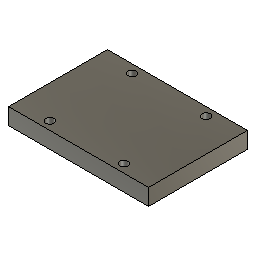
Top (Autodesk Fusion 360 design; units mm, degrees)
Autodesk Fusion 360 part; units mm, degrees
ref_plane "WorkPlane1" through (0, 0, 40) normal (0, 0, 1) x (1, 0, 0)
sketch "Sketch1" plane through (0, 0, 40) normal (0, 0, 1) x (1, 0, 0)
  line L0 (-10, 50) -> (75, 50)
  line L1 (75, 50) -> (75, -10)
  line L2 (75, -10) -> (-10, -10)
  line L3 (-10, -10) -> (-10, 50)
  constraint horizontal L0
  constraint vertical L1
  constraint horizontal L2
  constraint vertical L3
extrude "Extrude1" add sketch "Sketch1" along normal blind 10
sketch "Sketch2" plane through (0, 0, 50) normal (0, 0, 1) x (-1, 0, 0)
  line L0 (10, 10) -> (-75, 10)
  line L1 (-75, 10) -> (-75, -50)
  line L2 (-75, -50) -> (10, -50)
  line L3 (10, -50) -> (10, 10)
  circle A0 centre (-10, 5) radius 2.5
  circle A1 centre (-55, 5) radius 2.5
  circle A2 centre (-55, -45) radius 2.5
  circle A3 centre (-10, -45) radius 2.5
  dimension "d11" = 5
  dimension "d12" = 5
  dimension "d13" = 5
  dimension "d14" = 5
  measures "d11" diameter of A0
  measures "d12" diameter of A1
  measures "d13" diameter of A2
  measures "d14" diameter of A3
extrude "Extrude2" cut sketch "Sketch2" against normal blind 10 contours A0 | A1 | A2 | A3
